Autodesk Fusion 360 part; units mm, degrees
(part 2 of 2)
  line L907 (437.3348, -83.014) -> (451.1912, -83.014)
  line L908 (430.4066, -71.014) -> (437.3348, -83.014)
  line L909 (437.3348, -59.014) -> (430.4066, -71.014)
  line L910 (474.5739, -45.514) -> (460.7175, -45.514)
  line L911 (453.7893, -57.514) -> (460.7175, -69.514)
  line L912 (460.7175, -69.514) -> (474.5739, -69.514)
  line L913 (474.5739, -69.514) -> (481.5021, -57.514)
  line L914 (481.5021, -57.514) -> (474.5739, -45.514)
  line L915 (474.5739, -72.514) -> (460.7175, -72.514)
  line L916 (460.7175, -72.514) -> (453.7893, -84.514)
  line L917 (453.7893, -84.514) -> (460.7175, -96.514)
  line L918 (460.7175, -96.514) -> (474.5739, -96.514)
  line L919 (474.5739, -96.514) -> (481.5021, -84.514)
  line L920 (481.5021, -84.514) -> (474.5739, -72.514)
  line L921 (79.6636, 212.4814) -> (86.5918, 200.4814)
  line L922 (86.5918, 224.4814) -> (79.6636, 212.4814)
  line L923 (100.4482, 224.4814) -> (86.5918, 224.4814)
  line L924 (107.3764, 212.4814) -> (100.4482, 224.4814)
  line L925 (100.4482, 200.4814) -> (107.3764, 212.4814)
  line L926 (109.9745, 210.9814) -> (103.0463, 198.9814)
  line L927 (86.5918, 200.4814) -> (100.4482, 200.4814)
  line L928 (100.4482, 197.4814) -> (86.5918, 197.4814)
  line L929 (107.3764, 185.4814) -> (100.4482, 197.4814)
  line L930 (100.4482, 173.4814) -> (107.3764, 185.4814)
  line L931 (86.5918, 173.4814) -> (100.4482, 173.4814)
  line L932 (79.6636, 185.4814) -> (86.5918, 173.4814)
  line L933 (86.5918, 197.4814) -> (79.6636, 185.4814)
  line L934 (123.8309, 210.9814) -> (109.9745, 210.9814)
  line L935 (103.0463, 198.9814) -> (109.9745, 186.9814)
  line L936 (109.9745, 186.9814) -> (123.8309, 186.9814)
  line L937 (123.8309, 186.9814) -> (130.7591, 198.9814)
  line L938 (130.7591, 198.9814) -> (123.8309, 210.9814)
  line L939 (123.8309, 183.9814) -> (109.9745, 183.9814)
  line L940 (109.9745, 183.9814) -> (103.0463, 171.9814)
  line L941 (103.0463, 171.9814) -> (109.9745, 159.9814)
  line L942 (109.9745, 159.9814) -> (123.8309, 159.9814)
  line L943 (123.8309, 159.9814) -> (130.7591, 171.9814)
  line L944 (130.7591, 171.9814) -> (123.8309, 183.9814)
  line L945 (126.429, 185.4814) -> (133.3572, 173.4814)
  line L946 (133.3572, 197.4814) -> (126.429, 185.4814)
  line L947 (147.2136, 197.4814) -> (133.3572, 197.4814)
  line L948 (154.1418, 185.4814) -> (147.2136, 197.4814)
  line L949 (147.2136, 173.4814) -> (154.1418, 185.4814)
  line L950 (156.7399, 183.9814) -> (149.8117, 171.9814)
  line L951 (133.3572, 173.4814) -> (147.2136, 173.4814)
  line L952 (147.2136, 170.4814) -> (133.3572, 170.4814)
  line L953 (154.1418, 158.4814) -> (147.2136, 170.4814)
  line L954 (147.2136, 146.4814) -> (154.1418, 158.4814)
  line L955 (133.3572, 146.4814) -> (147.2136, 146.4814)
  line L956 (126.429, 158.4814) -> (133.3572, 146.4814)
  line L957 (133.3572, 170.4814) -> (126.429, 158.4814)
  line L958 (170.5963, 183.9814) -> (156.7399, 183.9814)
  line L959 (149.8117, 171.9814) -> (156.7399, 159.9814)
  line L960 (156.7399, 159.9814) -> (170.5963, 159.9814)
  line L961 (170.5963, 159.9814) -> (177.5245, 171.9814)
  line L962 (177.5245, 171.9814) -> (170.5963, 183.9814)
  line L963 (170.5963, 156.9814) -> (156.7399, 156.9814)
  line L964 (156.7399, 156.9814) -> (149.8117, 144.9814)
  line L965 (149.8117, 144.9814) -> (156.7399, 132.9814)
  line L966 (156.7399, 132.9814) -> (170.5963, 132.9814)
  line L967 (170.5963, 132.9814) -> (177.5245, 144.9814)
  line L968 (177.5245, 144.9814) -> (170.5963, 156.9814)
  line L969 (173.1943, 158.4814) -> (180.1225, 146.4814)
  line L970 (180.1225, 170.4814) -> (173.1943, 158.4814)
  line L971 (193.9789, 170.4814) -> (180.1225, 170.4814)
  line L972 (200.9072, 158.4814) -> (193.9789, 170.4814)
  line L973 (193.9789, 146.4814) -> (200.9072, 158.4814)
  line L974 (203.5052, 156.9814) -> (196.577, 144.9814)
  line L975 (180.1225, 146.4814) -> (193.9789, 146.4814)
  line L976 (193.9789, 143.4814) -> (180.1225, 143.4814)
  line L977 (200.9072, 131.4814) -> (193.9789, 143.4814)
  line L978 (193.9789, 119.4814) -> (200.9072, 131.4814)
  line L979 (180.1225, 119.4814) -> (193.9789, 119.4814)
  line L980 (173.1943, 131.4814) -> (180.1225, 119.4814)
  line L981 (180.1225, 143.4814) -> (173.1943, 131.4814)
  line L982 (217.3616, 156.9814) -> (203.5052, 156.9814)
  line L983 (196.577, 144.9814) -> (203.5052, 132.9814)
  line L984 (203.5052, 132.9814) -> (217.3616, 132.9814)
  line L985 (217.3616, 132.9814) -> (224.2898, 144.9814)
  line L986 (224.2898, 144.9814) -> (217.3616, 156.9814)
  line L987 (217.3616, 129.9814) -> (203.5052, 129.9814)
  line L988 (203.5052, 129.9814) -> (196.577, 117.9814)
  line L989 (196.577, 117.9814) -> (203.5052, 105.9814)
  line L990 (203.5052, 105.9814) -> (217.3616, 105.9814)
  line L991 (217.3616, 105.9814) -> (224.2898, 117.9814)
  line L992 (224.2898, 117.9814) -> (217.3616, 129.9814)
  line L993 (219.9597, 131.4814) -> (226.8879, 119.4814)
  line L994 (226.8879, 143.4814) -> (219.9597, 131.4814)
  line L995 (240.7443, 143.4814) -> (226.8879, 143.4814)
  line L996 (247.6725, 131.4814) -> (240.7443, 143.4814)
  line L997 (240.7443, 119.4814) -> (247.6725, 131.4814)
  line L998 (250.2706, 129.9814) -> (243.3424, 117.9814)
  line L999 (226.8879, 119.4814) -> (240.7443, 119.4814)
  line L1000 (240.7443, 116.4814) -> (226.8879, 116.4814)
  line L1001 (247.6725, 104.4814) -> (240.7443, 116.4814)
  line L1002 (240.7443, 92.4814) -> (247.6725, 104.4814)
  line L1003 (226.8879, 92.4814) -> (240.7443, 92.4814)
  line L1004 (219.9597, 104.4814) -> (226.8879, 92.4814)
  line L1005 (226.8879, 116.4814) -> (219.9597, 104.4814)
  line L1006 (264.127, 129.9814) -> (250.2706, 129.9814)
  line L1007 (243.3424, 117.9814) -> (250.2706, 105.9814)
  line L1008 (250.2706, 105.9814) -> (264.127, 105.9814)
  line L1009 (264.127, 105.9814) -> (271.0552, 117.9814)
  line L1010 (271.0552, 117.9814) -> (264.127, 129.9814)
  line L1011 (264.127, 102.9814) -> (250.2706, 102.9814)
  line L1012 (250.2706, 102.9814) -> (243.3424, 90.9814)
  line L1013 (243.3424, 90.9814) -> (250.2706, 78.9814)
  line L1014 (250.2706, 78.9814) -> (264.127, 78.9814)
  line L1015 (264.127, 78.9814) -> (271.0552, 90.9814)
  line L1016 (271.0552, 90.9814) -> (264.127, 102.9814)
  line L1017 (266.7251, 104.4814) -> (273.6533, 92.4814)
  line L1018 (273.6533, 116.4814) -> (266.7251, 104.4814)
  line L1019 (287.5097, 116.4814) -> (273.6533, 116.4814)
  line L1020 (294.4379, 104.4814) -> (287.5097, 116.4814)
  line L1021 (287.5097, 92.4814) -> (294.4379, 104.4814)
  line L1022 (297.036, 102.9814) -> (290.1078, 90.9814)
  line L1023 (273.6533, 92.4814) -> (287.5097, 92.4814)
  line L1024 (287.5097, 89.4814) -> (273.6533, 89.4814)
  line L1025 (294.4379, 77.4814) -> (287.5097, 89.4814)
  line L1026 (287.5097, 65.4814) -> (294.4379, 77.4814)
  line L1027 (273.6533, 65.4814) -> (287.5097, 65.4814)
  line L1028 (266.7251, 77.4814) -> (273.6533, 65.4814)
  line L1029 (273.6533, 89.4814) -> (266.7251, 77.4814)
  line L1030 (310.8924, 102.9814) -> (297.036, 102.9814)
  line L1031 (290.1078, 90.9814) -> (297.036, 78.9814)
  line L1032 (297.036, 78.9814) -> (310.8924, 78.9814)
  line L1033 (310.8924, 78.9814) -> (317.8206, 90.9814)
  line L1034 (317.8206, 90.9814) -> (310.8924, 102.9814)
  line L1035 (310.8924, 75.9814) -> (297.036, 75.9814)
  line L1036 (297.036, 75.9814) -> (290.1078, 63.9814)
  line L1037 (290.1078, 63.9814) -> (297.036, 51.9814)
  line L1038 (297.036, 51.9814) -> (310.8924, 51.9814)
  line L1039 (310.8924, 51.9814) -> (317.8206, 63.9814)
  line L1040 (317.8206, 63.9814) -> (310.8924, 75.9814)
  line L1041 (313.4905, 77.4814) -> (320.4187, 65.4814)
  line L1042 (320.4187, 89.4814) -> (313.4905, 77.4814)
  line L1043 (334.2751, 89.4814) -> (320.4187, 89.4814)
  line L1044 (341.2033, 77.4814) -> (334.2751, 89.4814)
  line L1045 (334.2751, 65.4814) -> (341.2033, 77.4814)
  line L1046 (343.8013, 75.9814) -> (336.8731, 63.9814)
  line L1047 (320.4187, 65.4814) -> (334.2751, 65.4814)
  line L1048 (334.2751, 62.4814) -> (320.4187, 62.4814)
  line L1049 (341.2033, 50.4814) -> (334.2751, 62.4814)
  line L1050 (334.2751, 38.4814) -> (341.2033, 50.4814)
  line L1051 (320.4187, 38.4814) -> (334.2751, 38.4814)
  line L1052 (313.4905, 50.4814) -> (320.4187, 38.4814)
  line L1053 (320.4187, 62.4814) -> (313.4905, 50.4814)
  line L1054 (357.6577, 75.9814) -> (343.8013, 75.9814)
  line L1055 (336.8731, 63.9814) -> (343.8013, 51.9814)
  line L1056 (343.8013, 51.9814) -> (357.6577, 51.9814)
  line L1057 (357.6577, 51.9814) -> (364.586, 63.9814)
  line L1058 (364.586, 63.9814) -> (357.6577, 75.9814)
  line L1059 (357.6577, 48.9814) -> (343.8013, 48.9814)
  line L1060 (343.8013, 48.9814) -> (336.8731, 36.9814)
  line L1061 (336.8731, 36.9814) -> (343.8013, 24.9814)
  line L1062 (343.8013, 24.9814) -> (357.6577, 24.9814)
  line L1063 (357.6577, 24.9814) -> (364.586, 36.9814)
  line L1064 (364.586, 36.9814) -> (357.6577, 48.9814)
  line L1065 (360.2558, 50.4814) -> (367.184, 38.4814)
  line L1066 (367.184, 62.4814) -> (360.2558, 50.4814)
  line L1067 (381.0404, 62.4814) -> (367.184, 62.4814)
  line L1068 (387.9686, 50.4814) -> (381.0404, 62.4814)
  line L1069 (381.0404, 38.4814) -> (387.9686, 50.4814)
  line L1070 (390.5667, 48.9814) -> (383.6385, 36.9814)
  line L1071 (367.184, 38.4814) -> (381.0404, 38.4814)
  line L1072 (381.0404, 35.4814) -> (367.184, 35.4814)
  line L1073 (387.9686, 23.4814) -> (381.0404, 35.4814)
  line L1074 (381.0404, 11.4814) -> (387.9686, 23.4814)
  line L1075 (367.184, 11.4814) -> (381.0404, 11.4814)
  line L1076 (360.2558, 23.4814) -> (367.184, 11.4814)
  line L1077 (367.184, 35.4814) -> (360.2558, 23.4814)
  line L1078 (404.4231, 48.9814) -> (390.5667, 48.9814)
  line L1079 (383.6385, 36.9814) -> (390.5667, 24.9814)
  line L1080 (390.5667, 24.9814) -> (404.4231, 24.9814)
  line L1081 (404.4231, 24.9814) -> (411.3513, 36.9814)
  line L1082 (411.3513, 36.9814) -> (404.4231, 48.9814)
  line L1083 (404.4231, 21.9814) -> (390.5667, 21.9814)
  line L1084 (390.5667, 21.9814) -> (383.6385, 9.9814)
  line L1085 (383.6385, 9.9814) -> (390.5667, -2.0186)
  line L1086 (390.5667, -2.0186) -> (404.4231, -2.0186)
  line L1087 (404.4231, -2.0186) -> (411.3513, 9.9814)
  line L1088 (411.3513, 9.9814) -> (404.4231, 21.9814)
  line L1089 (407.0212, 23.4814) -> (413.9494, 11.4814)
  line L1090 (413.9494, 35.4814) -> (407.0212, 23.4814)
  line L1091 (427.8058, 35.4814) -> (413.9494, 35.4814)
  line L1092 (434.734, 23.4814) -> (427.8058, 35.4814)
  line L1093 (427.8058, 11.4814) -> (434.734, 23.4814)
  line L1094 (437.3321, 21.9814) -> (430.4039, 9.9814)
  line L1095 (413.9494, 11.4814) -> (427.8058, 11.4814)
  line L1096 (427.8058, 8.4814) -> (413.9494, 8.4814)
  line L1097 (434.734, -3.5186) -> (427.8058, 8.4814)
  line L1098 (427.8058, -15.5186) -> (434.734, -3.5186)
  line L1099 (413.9494, -15.5186) -> (427.8058, -15.5186)
  line L1100 (407.0212, -3.5186) -> (413.9494, -15.5186)
  line L1101 (413.9494, 8.4814) -> (407.0212, -3.5186)
  line L1102 (451.1885, 21.9814) -> (437.3321, 21.9814)
  line L1103 (430.4039, 9.9814) -> (437.3321, -2.0186)
  line L1104 (437.3321, -2.0186) -> (451.1885, -2.0186)
  line L1105 (451.1885, -2.0186) -> (458.1167, 9.9814)
  line L1106 (458.1167, 9.9814) -> (451.1885, 21.9814)
  line L1107 (451.1885, -5.0186) -> (437.3321, -5.0186)
  line L1108 (437.3321, -5.0186) -> (430.4039, -17.0186)
  line L1109 (430.4039, -17.0186) -> (437.3321, -29.0186)
  line L1110 (437.3321, -29.0186) -> (451.1885, -29.0186)
  line L1111 (451.1885, -29.0186) -> (458.1167, -17.0186)
  line L1112 (458.1167, -17.0186) -> (451.1885, -5.0186)
  line L1113 (453.7866, -3.5186) -> (460.7148, -15.5186)
  line L1114 (460.7148, 8.4814) -> (453.7866, -3.5186)
  line L1115 (474.5712, 8.4814) -> (460.7148, 8.4814)
  line L1116 (481.4994, -3.5186) -> (474.5712, 8.4814)
  line L1117 (474.5712, -15.5186) -> (481.4994, -3.5186)
  line L1118 (484.0975, -5.0186) -> (477.1693, -17.0186)
  line L1119 (460.7148, -15.5186) -> (474.5712, -15.5186)
  line L1120 (474.5712, -18.5186) -> (460.7148, -18.5186)
  line L1121 (481.4994, -30.5186) -> (474.5712, -18.5186)
  line L1122 (474.5712, -42.5186) -> (481.4994, -30.5186)
  line L1123 (460.7148, -42.5186) -> (474.5712, -42.5186)
  line L1124 (453.7866, -30.5186) -> (460.7148, -42.5186)
  line L1125 (460.7148, -18.5186) -> (453.7866, -30.5186)
  line L1126 (497.9539, -5.0186) -> (484.0975, -5.0186)
  line L1127 (477.1693, -17.0186) -> (484.0975, -29.0186)
  line L1128 (484.0975, -29.0186) -> (497.9539, -29.0186)
  line L1129 (497.9539, -29.0186) -> (504.8821, -17.0186)
  line L1130 (504.8821, -17.0186) -> (497.9539, -5.0186)
  line L1131 (497.9539, -32.0186) -> (484.0975, -32.0186)
  line L1132 (484.0975, -32.0186) -> (477.1693, -44.0186)
  line L1133 (477.1693, -44.0186) -> (484.0975, -56.0186)
  line L1134 (484.0975, -56.0186) -> (497.9539, -56.0186)
  line L1135 (497.9539, -56.0186) -> (504.8821, -44.0186)
  line L1136 (504.8821, -44.0186) -> (497.9539, -32.0186)
  line L1137 (103.0436, 252.9767) -> (109.9718, 240.9767)
  line L1138 (109.9718, 264.9767) -> (103.0436, 252.9767)
  line L1139 (123.8282, 264.9767) -> (109.9718, 264.9767)
  line L1140 (130.7564, 252.9767) -> (123.8282, 264.9767)
  line L1141 (123.8282, 240.9767) -> (130.7564, 252.9767)
  line L1142 (133.3545, 251.4767) -> (126.4263, 239.4767)
  line L1143 (109.9718, 240.9767) -> (123.8282, 240.9767)
  line L1144 (123.8282, 237.9767) -> (109.9718, 237.9767)
  line L1145 (130.7564, 225.9767) -> (123.8282, 237.9767)
  line L1146 (123.8282, 213.9767) -> (130.7564, 225.9767)
  line L1147 (109.9718, 213.9767) -> (123.8282, 213.9767)
  line L1148 (103.0436, 225.9767) -> (109.9718, 213.9767)
  line L1149 (109.9718, 237.9767) -> (103.0436, 225.9767)
  line L1150 (147.2109, 251.4767) -> (133.3545, 251.4767)
  line L1151 (126.4263, 239.4767) -> (133.3545, 227.4767)
  line L1152 (133.3545, 227.4767) -> (147.2109, 227.4767)
  line L1153 (147.2109, 227.4767) -> (154.1391, 239.4767)
  line L1154 (154.1391, 239.4767) -> (147.2109, 251.4767)
  line L1155 (147.2109, 224.4767) -> (133.3545, 224.4767)
  line L1156 (133.3545, 224.4767) -> (126.4263, 212.4767)
  line L1157 (126.4263, 212.4767) -> (133.3545, 200.4767)
  line L1158 (133.3545, 200.4767) -> (147.2109, 200.4767)
  line L1159 (147.2109, 200.4767) -> (154.1391, 212.4767)
  line L1160 (154.1391, 212.4767) -> (147.2109, 224.4767)
  line L1161 (149.809, 225.9767) -> (156.7372, 213.9767)
  line L1162 (156.7372, 237.9767) -> (149.809, 225.9767)
  line L1163 (170.5936, 237.9767) -> (156.7372, 237.9767)
  line L1164 (177.5218, 225.9767) -> (170.5936, 237.9767)
  line L1165 (170.5936, 213.9767) -> (177.5218, 225.9767)
  line L1166 (180.1199, 224.4767) -> (173.1917, 212.4767)
  line L1167 (156.7372, 213.9767) -> (170.5936, 213.9767)
  line L1168 (170.5936, 210.9767) -> (156.7372, 210.9767)
  line L1169 (177.5218, 198.9767) -> (170.5936, 210.9767)
  line L1170 (170.5936, 186.9767) -> (177.5218, 198.9767)
  line L1171 (156.7372, 186.9767) -> (170.5936, 186.9767)
  line L1172 (149.809, 198.9767) -> (156.7372, 186.9767)
  line L1173 (156.7372, 210.9767) -> (149.809, 198.9767)
  line L1174 (193.9763, 224.4767) -> (180.1199, 224.4767)
  line L1175 (173.1917, 212.4767) -> (180.1199, 200.4767)
  line L1176 (180.1199, 200.4767) -> (193.9763, 200.4767)
  line L1177 (193.9763, 200.4767) -> (200.9045, 212.4767)
  line L1178 (200.9045, 212.4767) -> (193.9763, 224.4767)
  line L1179 (193.9763, 197.4767) -> (180.1199, 197.4767)
  line L1180 (180.1199, 197.4767) -> (173.1917, 185.4767)
  line L1181 (173.1917, 185.4767) -> (180.1199, 173.4767)
  line L1182 (180.1199, 173.4767) -> (193.9763, 173.4767)
  line L1183 (193.9763, 173.4767) -> (200.9045, 185.4767)
  line L1184 (200.9045, 185.4767) -> (193.9763, 197.4767)
  line L1185 (196.5743, 198.9767) -> (203.5025, 186.9767)
  line L1186 (203.5025, 210.9767) -> (196.5743, 198.9767)
  line L1187 (217.3589, 210.9767) -> (203.5025, 210.9767)
  line L1188 (224.2872, 198.9767) -> (217.3589, 210.9767)
  line L1189 (217.3589, 186.9767) -> (224.2872, 198.9767)
  line L1190 (226.8852, 197.4767) -> (219.957, 185.4767)
  line L1191 (203.5025, 186.9767) -> (217.3589, 186.9767)
  line L1192 (217.3589, 183.9767) -> (203.5025, 183.9767)
  line L1193 (224.2872, 171.9767) -> (217.3589, 183.9767)
  line L1194 (217.3589, 159.9767) -> (224.2872, 171.9767)
  line L1195 (203.5025, 159.9767) -> (217.3589, 159.9767)
  line L1196 (196.5743, 171.9767) -> (203.5025, 159.9767)
  line L1197 (203.5025, 183.9767) -> (196.5743, 171.9767)
  line L1198 (240.7416, 197.4767) -> (226.8852, 197.4767)
  line L1199 (219.957, 185.4767) -> (226.8852, 173.4767)
  line L1200 (226.8852, 173.4767) -> (240.7416, 173.4767)
  line L1201 (240.7416, 173.4767) -> (247.6698, 185.4767)
  line L1202 (247.6698, 185.4767) -> (240.7416, 197.4767)
  line L1203 (240.7416, 170.4767) -> (226.8852, 170.4767)
  line L1204 (226.8852, 170.4767) -> (219.957, 158.4767)
  line L1205 (219.957, 158.4767) -> (226.8852, 146.4767)
  line L1206 (226.8852, 146.4767) -> (240.7416, 146.4767)
  line L1207 (240.7416, 146.4767) -> (247.6698, 158.4767)
  line L1208 (247.6698, 158.4767) -> (240.7416, 170.4767)
  line L1209 (243.3397, 171.9767) -> (250.2679, 159.9767)
  line L1210 (250.2679, 183.9767) -> (243.3397, 171.9767)
  line L1211 (264.1243, 183.9767) -> (250.2679, 183.9767)
  line L1212 (271.0525, 171.9767) -> (264.1243, 183.9767)
  line L1213 (264.1243, 159.9767) -> (271.0525, 171.9767)
  line L1214 (273.6506, 170.4767) -> (266.7224, 158.4767)
  line L1215 (250.2679, 159.9767) -> (264.1243, 159.9767)
  line L1216 (264.1243, 156.9767) -> (250.2679, 156.9767)
  line L1217 (271.0525, 144.9767) -> (264.1243, 156.9767)
  line L1218 (264.1243, 132.9767) -> (271.0525, 144.9767)
  line L1219 (250.2679, 132.9767) -> (264.1243, 132.9767)
  line L1220 (243.3397, 144.9767) -> (250.2679, 132.9767)
  line L1221 (250.2679, 156.9767) -> (243.3397, 144.9767)
  line L1222 (287.507, 170.4767) -> (273.6506, 170.4767)
  line L1223 (266.7224, 158.4767) -> (273.6506, 146.4767)
  line L1224 (273.6506, 146.4767) -> (287.507, 146.4767)
  line L1225 (287.507, 146.4767) -> (294.4352, 158.4767)
  line L1226 (294.4352, 158.4767) -> (287.507, 170.4767)
  line L1227 (287.507, 143.4767) -> (273.6506, 143.4767)
  line L1228 (273.6506, 143.4767) -> (266.7224, 131.4767)
  line L1229 (266.7224, 131.4767) -> (273.6506, 119.4767)
  line L1230 (273.6506, 119.4767) -> (287.507, 119.4767)
  line L1231 (287.507, 119.4767) -> (294.4352, 131.4767)
  line L1232 (294.4352, 131.4767) -> (287.507, 143.4767)
  line L1233 (290.1051, 144.9767) -> (297.0333, 132.9767)
  line L1234 (297.0333, 156.9767) -> (290.1051, 144.9767)
  line L1235 (310.8897, 156.9767) -> (297.0333, 156.9767)
  line L1236 (317.8179, 144.9767) -> (310.8897, 156.9767)
  line L1237 (310.8897, 132.9767) -> (317.8179, 144.9767)
  line L1238 (320.416, 143.4767) -> (313.4878, 131.4767)
  line L1239 (297.0333, 132.9767) -> (310.8897, 132.9767)
  line L1240 (310.8897, 129.9767) -> (297.0333, 129.9767)
  line L1241 (317.8179, 117.9767) -> (310.8897, 129.9767)
  line L1242 (310.8897, 105.9767) -> (317.8179, 117.9767)
  line L1243 (297.0333, 105.9767) -> (310.8897, 105.9767)
  line L1244 (290.1051, 117.9767) -> (297.0333, 105.9767)
  line L1245 (297.0333, 129.9767) -> (290.1051, 117.9767)
  line L1246 (334.2724, 143.4767) -> (320.416, 143.4767)
  line L1247 (313.4878, 131.4767) -> (320.416, 119.4767)
  line L1248 (320.416, 119.4767) -> (334.2724, 119.4767)
  line L1249 (334.2724, 119.4767) -> (341.2006, 131.4767)
  line L1250 (341.2006, 131.4767) -> (334.2724, 143.4767)
  line L1251 (334.2724, 116.4767) -> (320.416, 116.4767)
  line L1252 (320.416, 116.4767) -> (313.4878, 104.4767)
  line L1253 (313.4878, 104.4767) -> (320.416, 92.4767)
  line L1254 (320.416, 92.4767) -> (334.2724, 92.4767)
  line L1255 (334.2724, 92.4767) -> (341.2006, 104.4767)
  line L1256 (341.2006, 104.4767) -> (334.2724, 116.4767)
  line L1257 (336.8705, 117.9767) -> (343.7987, 105.9767)
  line L1258 (343.7987, 129.9767) -> (336.8705, 117.9767)
  line L1259 (357.6551, 129.9767) -> (343.7987, 129.9767)
  line L1260 (364.5833, 117.9767) -> (357.6551, 129.9767)
  line L1261 (357.6551, 105.9767) -> (364.5833, 117.9767)
  line L1262 (367.1813, 116.4767) -> (360.2531, 104.4767)
  line L1263 (343.7987, 105.9767) -> (357.6551, 105.9767)
  line L1264 (357.6551, 102.9767) -> (343.7987, 102.9767)
  line L1265 (364.5833, 90.9767) -> (357.6551, 102.9767)
  line L1266 (357.6551, 78.9767) -> (364.5833, 90.9767)
  line L1267 (343.7987, 78.9767) -> (357.6551, 78.9767)
  line L1268 (336.8705, 90.9767) -> (343.7987, 78.9767)
  line L1269 (343.7987, 102.9767) -> (336.8705, 90.9767)
  line L1270 (381.0377, 116.4767) -> (367.1813, 116.4767)
  line L1271 (360.2531, 104.4767) -> (367.1813, 92.4767)
  line L1272 (367.1813, 92.4767) -> (381.0377, 92.4767)
  line L1273 (381.0377, 92.4767) -> (387.966, 104.4767)
  line L1274 (387.966, 104.4767) -> (381.0377, 116.4767)
  line L1275 (381.0377, 89.4767) -> (367.1813, 89.4767)
  line L1276 (367.1813, 89.4767) -> (360.2531, 77.4767)
  line L1277 (360.2531, 77.4767) -> (367.1813, 65.4767)
  line L1278 (367.1813, 65.4767) -> (381.0377, 65.4767)
  line L1279 (381.0377, 65.4767) -> (387.966, 77.4767)
  line L1280 (387.966, 77.4767) -> (381.0377, 89.4767)
  line L1281 (383.6358, 90.9767) -> (390.564, 78.9767)
  line L1282 (390.564, 102.9767) -> (383.6358, 90.9767)
  line L1283 (404.4204, 102.9767) -> (390.564, 102.9767)
  line L1284 (411.3486, 90.9767) -> (404.4204, 102.9767)
  line L1285 (404.4204, 78.9767) -> (411.3486, 90.9767)
  line L1286 (413.9467, 89.4767) -> (407.0185, 77.4767)
  line L1287 (390.564, 78.9767) -> (404.4204, 78.9767)
  line L1288 (404.4204, 75.9767) -> (390.564, 75.9767)
  line L1289 (411.3486, 63.9767) -> (404.4204, 75.9767)
  line L1290 (404.4204, 51.9767) -> (411.3486, 63.9767)
  line L1291 (390.564, 51.9767) -> (404.4204, 51.9767)
  line L1292 (383.6358, 63.9767) -> (390.564, 51.9767)
  line L1293 (390.564, 75.9767) -> (383.6358, 63.9767)
  line L1294 (427.8031, 89.4767) -> (413.9467, 89.4767)
  line L1295 (407.0185, 77.4767) -> (413.9467, 65.4767)
  line L1296 (413.9467, 65.4767) -> (427.8031, 65.4767)
  line L1297 (427.8031, 65.4767) -> (434.7313, 77.4767)
  line L1298 (434.7313, 77.4767) -> (427.8031, 89.4767)
  line L1299 (427.8031, 62.4767) -> (413.9467, 62.4767)
  line L1300 (413.9467, 62.4767) -> (407.0185, 50.4767)
  line L1301 (407.0185, 50.4767) -> (413.9467, 38.4767)
  line L1302 (413.9467, 38.4767) -> (427.8031, 38.4767)
  line L1303 (427.8031, 38.4767) -> (434.7313, 50.4767)
  line L1304 (434.7313, 50.4767) -> (427.8031, 62.4767)
  line L1305 (430.4012, 63.9767) -> (437.3294, 51.9767)
  line L1306 (437.3294, 75.9767) -> (430.4012, 63.9767)
  line L1307 (451.1858, 75.9767) -> (437.3294, 75.9767)
  line L1308 (458.114, 63.9767) -> (451.1858, 75.9767)
  line L1309 (451.1858, 51.9767) -> (458.114, 63.9767)
  line L1310 (460.7121, 62.4767) -> (453.7839, 50.4767)
  line L1311 (437.3294, 51.9767) -> (451.1858, 51.9767)
  line L1312 (451.1858, 48.9767) -> (437.3294, 48.9767)
  line L1313 (458.114, 36.9767) -> (451.1858, 48.9767)
  line L1314 (451.1858, 24.9767) -> (458.114, 36.9767)
  line L1315 (437.3294, 24.9767) -> (451.1858, 24.9767)
  line L1316 (430.4012, 36.9767) -> (437.3294, 24.9767)
  line L1317 (437.3294, 48.9767) -> (430.4012, 36.9767)
  line L1318 (474.5685, 62.4767) -> (460.7121, 62.4767)
  line L1319 (453.7839, 50.4767) -> (460.7121, 38.4767)
  line L1320 (460.7121, 38.4767) -> (474.5685, 38.4767)
  line L1321 (474.5685, 38.4767) -> (481.4967, 50.4767)
  line L1322 (481.4967, 50.4767) -> (474.5685, 62.4767)
  line L1323 (474.5685, 35.4767) -> (460.7121, 35.4767)
  line L1324 (460.7121, 35.4767) -> (453.7839, 23.4767)
  line L1325 (453.7839, 23.4767) -> (460.7121, 11.4767)
  line L1326 (460.7121, 11.4767) -> (474.5685, 11.4767)
  line L1327 (474.5685, 11.4767) -> (481.4967, 23.4767)
  line L1328 (481.4967, 23.4767) -> (474.5685, 35.4767)
  line L1329 (477.1666, 36.9767) -> (484.0948, 24.9767)
  line L1330 (484.0948, 48.9767) -> (477.1666, 36.9767)
  line L1331 (497.9512, 48.9767) -> (484.0948, 48.9767)
  line L1332 (504.8794, 36.9767) -> (497.9512, 48.9767)
  line L1333 (497.9512, 24.9767) -> (504.8794, 36.9767)
  line L1334 (507.4775, 35.4767) -> (500.5493, 23.4767)
  line L1335 (484.0948, 24.9767) -> (497.9512, 24.9767)
  line L1336 (497.9512, 21.9767) -> (484.0948, 21.9767)
  line L1337 (504.8794, 9.9767) -> (497.9512, 21.9767)
  line L1338 (497.9512, -2.0233) -> (504.8794, 9.9767)
  line L1339 (484.0948, -2.0233) -> (497.9512, -2.0233)
  line L1340 (477.1666, 9.9767) -> (484.0948, -2.0233)
  line L1341 (484.0948, 21.9767) -> (477.1666, 9.9767)
  line L1342 (521.3339, 35.4767) -> (507.4775, 35.4767)
  line L1343 (500.5493, 23.4767) -> (507.4775, 11.4767)
  line L1344 (507.4775, 11.4767) -> (521.3339, 11.4767)
  line L1345 (521.3339, 11.4767) -> (528.2621, 23.4767)
  line L1346 (528.2621, 23.4767) -> (521.3339, 35.4767)
  line L1347 (521.3339, 8.4767) -> (507.4775, 8.4767)
  line L1348 (507.4775, 8.4767) -> (500.5493, -3.5233)
  line L1349 (500.5493, -3.5233) -> (507.4775, -15.5233)
  line L1350 (507.4775, -15.5233) -> (521.3339, -15.5233)
  line L1351 (521.3339, -15.5233) -> (528.2621, -3.5233)
  line L1352 (528.2621, -3.5233) -> (521.3339, 8.4767)
  line L1353 (126.4236, 293.4721) -> (133.3518, 281.4721)
  line L1354 (133.3518, 305.4721) -> (126.4236, 293.4721)
  line L1355 (147.2082, 305.4721) -> (133.3518, 305.4721)
  line L1356 (154.1364, 293.4721) -> (147.2082, 305.4721)
  line L1357 (147.2082, 281.4721) -> (154.1364, 293.4721)
  line L1358 (156.7345, 291.9721) -> (149.8063, 279.9721)
  line L1359 (133.3518, 281.4721) -> (147.2082, 281.4721)
  line L1360 (147.2082, 278.4721) -> (133.3518, 278.4721)
  line L1361 (154.1364, 266.4721) -> (147.2082, 278.4721)
  line L1362 (147.2082, 254.4721) -> (154.1364, 266.4721)
  line L1363 (133.3518, 254.4721) -> (147.2082, 254.4721)
  line L1364 (126.4236, 266.4721) -> (133.3518, 254.4721)
  line L1365 (133.3518, 278.4721) -> (126.4236, 266.4721)
  line L1366 (170.5909, 291.9721) -> (156.7345, 291.9721)
  line L1367 (149.8063, 279.9721) -> (156.7345, 267.9721)
  line L1368 (156.7345, 267.9721) -> (170.5909, 267.9721)
  line L1369 (170.5909, 267.9721) -> (177.5191, 279.9721)
  line L1370 (177.5191, 279.9721) -> (170.5909, 291.9721)
  line L1371 (170.5909, 264.9721) -> (156.7345, 264.9721)
  line L1372 (156.7345, 264.9721) -> (149.8063, 252.9721)
  line L1373 (149.8063, 252.9721) -> (156.7345, 240.9721)
  line L1374 (156.7345, 240.9721) -> (170.5909, 240.9721)
  line L1375 (170.5909, 240.9721) -> (177.5191, 252.9721)
  line L1376 (177.5191, 252.9721) -> (170.5909, 264.9721)
  line L1377 (173.189, 266.4721) -> (180.1172, 254.4721)
  line L1378 (180.1172, 278.4721) -> (173.189, 266.4721)
  line L1379 (193.9736, 278.4721) -> (180.1172, 278.4721)
  line L1380 (200.9018, 266.4721) -> (193.9736, 278.4721)
  line L1381 (193.9736, 254.4721) -> (200.9018, 266.4721)
  line L1382 (203.4999, 264.9721) -> (196.5717, 252.9721)
  line L1383 (180.1172, 254.4721) -> (193.9736, 254.4721)
  line L1384 (193.9736, 251.4721) -> (180.1172, 251.4721)
  line L1385 (200.9018, 239.4721) -> (193.9736, 251.4721)
  line L1386 (193.9736, 227.4721) -> (200.9018, 239.4721)
  line L1387 (180.1172, 227.4721) -> (193.9736, 227.4721)
  line L1388 (173.189, 239.4721) -> (180.1172, 227.4721)
  line L1389 (180.1172, 251.4721) -> (173.189, 239.4721)
  line L1390 (217.3563, 264.9721) -> (203.4999, 264.9721)
  line L1391 (196.5717, 252.9721) -> (203.4999, 240.9721)
  line L1392 (203.4999, 240.9721) -> (217.3563, 240.9721)
  line L1393 (217.3563, 240.9721) -> (224.2845, 252.9721)
  line L1394 (224.2845, 252.9721) -> (217.3563, 264.9721)
  line L1395 (217.3563, 237.9721) -> (203.4999, 237.9721)
  line L1396 (203.4999, 237.9721) -> (196.5717, 225.9721)
  line L1397 (196.5717, 225.9721) -> (203.4999, 213.9721)
  line L1398 (203.4999, 213.9721) -> (217.3563, 213.9721)
  line L1399 (217.3563, 213.9721) -> (224.2845, 225.9721)
  line L1400 (224.2845, 225.9721) -> (217.3563, 237.9721)
  line L1401 (219.9543, 239.4721) -> (226.8825, 227.4721)
  line L1402 (226.8825, 251.4721) -> (219.9543, 239.4721)
  line L1403 (240.7389, 251.4721) -> (226.8825, 251.4721)
  line L1404 (247.6672, 239.4721) -> (240.7389, 251.4721)
  line L1405 (240.7389, 227.4721) -> (247.6672, 239.4721)
  line L1406 (250.2652, 237.9721) -> (243.337, 225.9721)
  line L1407 (226.8825, 227.4721) -> (240.7389, 227.4721)
  line L1408 (240.7389, 224.4721) -> (226.8825, 224.4721)
  line L1409 (247.6672, 212.4721) -> (240.7389, 224.4721)
  line L1410 (240.7389, 200.4721) -> (247.6672, 212.4721)
  line L1411 (226.8825, 200.4721) -> (240.7389, 200.4721)
  line L1412 (219.9543, 212.4721) -> (226.8825, 200.4721)
  line L1413 (226.8825, 224.4721) -> (219.9543, 212.4721)
  line L1414 (264.1216, 237.9721) -> (250.2652, 237.9721)
  line L1415 (243.337, 225.9721) -> (250.2652, 213.9721)
  line L1416 (250.2652, 213.9721) -> (264.1216, 213.9721)
  line L1417 (264.1216, 213.9721) -> (271.0498, 225.9721)
  line L1418 (271.0498, 225.9721) -> (264.1216, 237.9721)
  line L1419 (264.1216, 210.9721) -> (250.2652, 210.9721)
  line L1420 (250.2652, 210.9721) -> (243.337, 198.9721)
  line L1421 (243.337, 198.9721) -> (250.2652, 186.9721)
  line L1422 (250.2652, 186.9721) -> (264.1216, 186.9721)
  line L1423 (264.1216, 186.9721) -> (271.0498, 198.9721)
  line L1424 (271.0498, 198.9721) -> (264.1216, 210.9721)
  line L1425 (266.7197, 212.4721) -> (273.6479, 200.4721)
  line L1426 (273.6479, 224.4721) -> (266.7197, 212.4721)
  line L1427 (287.5043, 224.4721) -> (273.6479, 224.4721)
  line L1428 (294.4325, 212.4721) -> (287.5043, 224.4721)
  line L1429 (287.5043, 200.4721) -> (294.4325, 212.4721)
  line L1430 (297.0306, 210.9721) -> (290.1024, 198.9721)
  line L1431 (273.6479, 200.4721) -> (287.5043, 200.4721)
  line L1432 (287.5043, 197.4721) -> (273.6479, 197.4721)
  line L1433 (294.4325, 185.4721) -> (287.5043, 197.4721)
  line L1434 (287.5043, 173.4721) -> (294.4325, 185.4721)
  line L1435 (273.6479, 173.4721) -> (287.5043, 173.4721)
  line L1436 (266.7197, 185.4721) -> (273.6479, 173.4721)
  line L1437 (273.6479, 197.4721) -> (266.7197, 185.4721)
  line L1438 (310.887, 210.9721) -> (297.0306, 210.9721)
  line L1439 (290.1024, 198.9721) -> (297.0306, 186.9721)
  line L1440 (297.0306, 186.9721) -> (310.887, 186.9721)
  line L1441 (310.887, 186.9721) -> (317.8152, 198.9721)
  line L1442 (317.8152, 198.9721) -> (310.887, 210.9721)
  line L1443 (310.887, 183.9721) -> (297.0306, 183.9721)
  line L1444 (297.0306, 183.9721) -> (290.1024, 171.9721)
  line L1445 (290.1024, 171.9721) -> (297.0306, 159.9721)
  line L1446 (297.0306, 159.9721) -> (310.887, 159.9721)
  line L1447 (310.887, 159.9721) -> (317.8152, 171.9721)
  line L1448 (317.8152, 171.9721) -> (310.887, 183.9721)
  line L1449 (313.4851, 185.4721) -> (320.4133, 173.4721)
  line L1450 (320.4133, 197.4721) -> (313.4851, 185.4721)
  line L1451 (334.2697, 197.4721) -> (320.4133, 197.4721)
  line L1452 (341.1979, 185.4721) -> (334.2697, 197.4721)
  line L1453 (334.2697, 173.4721) -> (341.1979, 185.4721)
  line L1454 (343.796, 183.9721) -> (336.8678, 171.9721)
  line L1455 (320.4133, 173.4721) -> (334.2697, 173.4721)
  line L1456 (334.2697, 170.4721) -> (320.4133, 170.4721)
  line L1457 (341.1979, 158.4721) -> (334.2697, 170.4721)
  line L1458 (334.2697, 146.4721) -> (341.1979, 158.4721)
  line L1459 (320.4133, 146.4721) -> (334.2697, 146.4721)
  line L1460 (313.4851, 158.4721) -> (320.4133, 146.4721)
  line L1461 (320.4133, 170.4721) -> (313.4851, 158.4721)
  line L1462 (357.6524, 183.9721) -> (343.796, 183.9721)
  line L1463 (336.8678, 171.9721) -> (343.796, 159.9721)
  line L1464 (343.796, 159.9721) -> (357.6524, 159.9721)
  line L1465 (357.6524, 159.9721) -> (364.5806, 171.9721)
  line L1466 (364.5806, 171.9721) -> (357.6524, 183.9721)
  line L1467 (357.6524, 156.9721) -> (343.796, 156.9721)
  line L1468 (343.796, 156.9721) -> (336.8678, 144.9721)
  line L1469 (336.8678, 144.9721) -> (343.796, 132.9721)
  line L1470 (343.796, 132.9721) -> (357.6524, 132.9721)
  line L1471 (357.6524, 132.9721) -> (364.5806, 144.9721)
  line L1472 (364.5806, 144.9721) -> (357.6524, 156.9721)
  line L1473 (360.2505, 158.4721) -> (367.1787, 146.4721)
  line L1474 (367.1787, 170.4721) -> (360.2505, 158.4721)
  line L1475 (381.0351, 170.4721) -> (367.1787, 170.4721)
  line L1476 (387.9633, 158.4721) -> (381.0351, 170.4721)
  line L1477 (381.0351, 146.4721) -> (387.9633, 158.4721)
  line L1478 (390.5613, 156.9721) -> (383.6331, 144.9721)
  line L1479 (367.1787, 146.4721) -> (381.0351, 146.4721)
  line L1480 (381.0351, 143.4721) -> (367.1787, 143.4721)
  line L1481 (387.9633, 131.4721) -> (381.0351, 143.4721)
  line L1482 (381.0351, 119.4721) -> (387.9633, 131.4721)
  line L1483 (367.1787, 119.4721) -> (381.0351, 119.4721)
  line L1484 (360.2505, 131.4721) -> (367.1787, 119.4721)
  line L1485 (367.1787, 143.4721) -> (360.2505, 131.4721)
  line L1486 (404.4177, 156.9721) -> (390.5613, 156.9721)
  line L1487 (383.6331, 144.9721) -> (390.5613, 132.9721)
  line L1488 (390.5613, 132.9721) -> (404.4177, 132.9721)
  line L1489 (404.4177, 132.9721) -> (411.346, 144.9721)
  line L1490 (411.346, 144.9721) -> (404.4177, 156.9721)
  line L1491 (404.4177, 129.9721) -> (390.5613, 129.9721)
  line L1492 (390.5613, 129.9721) -> (383.6331, 117.9721)
  line L1493 (383.6331, 117.9721) -> (390.5613, 105.9721)
  line L1494 (390.5613, 105.9721) -> (404.4177, 105.9721)
  line L1495 (404.4177, 105.9721) -> (411.346, 117.9721)
  line L1496 (411.346, 117.9721) -> (404.4177, 129.9721)
  line L1497 (407.0158, 131.4721) -> (413.944, 119.4721)
  line L1498 (413.944, 143.4721) -> (407.0158, 131.4721)
  line L1499 (427.8004, 143.4721) -> (413.944, 143.4721)
  line L1500 (434.7286, 131.4721) -> (427.8004, 143.4721)
  line L1501 (427.8004, 119.4721) -> (434.7286, 131.4721)
  line L1502 (437.3267, 129.9721) -> (430.3985, 117.9721)
  line L1503 (413.944, 119.4721) -> (427.8004, 119.4721)
  line L1504 (427.8004, 116.4721) -> (413.944, 116.4721)
  line L1505 (434.7286, 104.4721) -> (427.8004, 116.4721)
  line L1506 (427.8004, 92.4721) -> (434.7286, 104.4721)
  line L1507 (413.944, 92.4721) -> (427.8004, 92.4721)
  line L1508 (407.0158, 104.4721) -> (413.944, 92.4721)
  line L1509 (413.944, 116.4721) -> (407.0158, 104.4721)
  line L1510 (451.1831, 129.9721) -> (437.3267, 129.9721)
  line L1511 (430.3985, 117.9721) -> (437.3267, 105.9721)
  line L1512 (437.3267, 105.9721) -> (451.1831, 105.9721)
  line L1513 (451.1831, 105.9721) -> (458.1113, 117.9721)
  line L1514 (458.1113, 117.9721) -> (451.1831, 129.9721)
  line L1515 (451.1831, 102.9721) -> (437.3267, 102.9721)
  line L1516 (437.3267, 102.9721) -> (430.3985, 90.9721)
  line L1517 (430.3985, 90.9721) -> (437.3267, 78.9721)
  line L1518 (437.3267, 78.9721) -> (451.1831, 78.9721)
  line L1519 (451.1831, 78.9721) -> (458.1113, 90.9721)
  line L1520 (458.1113, 90.9721) -> (451.1831, 102.9721)
  line L1521 (453.7812, 104.4721) -> (460.7094, 92.4721)
  line L1522 (460.7094, 116.4721) -> (453.7812, 104.4721)
  line L1523 (474.5658, 116.4721) -> (460.7094, 116.4721)
  line L1524 (481.494, 104.4721) -> (474.5658, 116.4721)
  line L1525 (474.5658, 92.4721) -> (481.494, 104.4721)
  line L1526 (484.0921, 102.9721) -> (477.1639, 90.9721)
  line L1527 (460.7094, 92.4721) -> (474.5658, 92.4721)
  line L1528 (474.5658, 89.4721) -> (460.7094, 89.4721)
  line L1529 (481.494, 77.4721) -> (474.5658, 89.4721)
  line L1530 (474.5658, 65.4721) -> (481.494, 77.4721)
  line L1531 (460.7094, 65.4721) -> (474.5658, 65.4721)
  line L1532 (453.7812, 77.4721) -> (460.7094, 65.4721)
  line L1533 (460.7094, 89.4721) -> (453.7812, 77.4721)
  line L1534 (497.9485, 102.9721) -> (484.0921, 102.9721)
  line L1535 (477.1639, 90.9721) -> (484.0921, 78.9721)
  line L1536 (484.0921, 78.9721) -> (497.9485, 78.9721)
  line L1537 (497.9485, 78.9721) -> (504.8767, 90.9721)
  line L1538 (504.8767, 90.9721) -> (497.9485, 102.9721)
  line L1539 (497.9485, 75.9721) -> (484.0921, 75.9721)
  line L1540 (484.0921, 75.9721) -> (477.1639, 63.9721)
  line L1541 (477.1639, 63.9721) -> (484.0921, 51.9721)
  line L1542 (484.0921, 51.9721) -> (497.9485, 51.9721)
  line L1543 (497.9485, 51.9721) -> (504.8767, 63.9721)
  line L1544 (504.8767, 63.9721) -> (497.9485, 75.9721)
  line L1545 (500.5466, 77.4721) -> (507.4748, 65.4721)
  line L1546 (507.4748, 89.4721) -> (500.5466, 77.4721)
  line L1547 (521.3312, 89.4721) -> (507.4748, 89.4721)
  line L1548 (528.2594, 77.4721) -> (521.3312, 89.4721)
  line L1549 (521.3312, 65.4721) -> (528.2594, 77.4721)
  line L1550 (530.8575, 75.9721) -> (523.9293, 63.9721)
  line L1551 (507.4748, 65.4721) -> (521.3312, 65.4721)
  line L1552 (521.3312, 62.4721) -> (507.4748, 62.4721)
  line L1553 (528.2594, 50.4721) -> (521.3312, 62.4721)
  line L1554 (521.3312, 38.4721) -> (528.2594, 50.4721)
  line L1555 (507.4748, 38.4721) -> (521.3312, 38.4721)
  line L1556 (500.5466, 50.4721) -> (507.4748, 38.4721)
  line L1557 (507.4748, 62.4721) -> (500.5466, 50.4721)
  line L1558 (544.7139, 75.9721) -> (530.8575, 75.9721)
  line L1559 (523.9293, 63.9721) -> (530.8575, 51.9721)
  line L1560 (530.8575, 51.9721) -> (544.7139, 51.9721)
  line L1561 (544.7139, 51.9721) -> (551.6421, 63.9721)
  line L1562 (551.6421, 63.9721) -> (544.7139, 75.9721)
  line L1563 (544.7139, 48.9721) -> (530.8575, 48.9721)
  line L1564 (530.8575, 48.9721) -> (523.9293, 36.9721)
  line L1565 (523.9293, 36.9721) -> (530.8575, 24.9721)
  line L1566 (530.8575, 24.9721) -> (544.7139, 24.9721)
  line L1567 (544.7139, 24.9721) -> (551.6421, 36.9721)
  line L1568 (551.6421, 36.9721) -> (544.7139, 48.9721)
  point P0 (340, 0)
  point P1 (150, 99.7133)
  point P2 (0, 50.5)
  point P3 (23.3827, 37)
  point P4 (0, 23.5)
  point P5 (23.3827, 10)
  point P6 (23.3827, 37)
  point P7 (0, 50.5)
  point P8 (23.3827, 37)
  point P9 (0, 23.5)
  point P10 (23.3827, 10)
  point P11 (0, 77.5)
  point P12 (137.5, 146)
  dimension "d1" = 490
  dimension "d10" = 20
  dimension "d11" = 20
  dimension "d12" = 20
  dimension "d13" = 20
  dimension "d16" = 4.35
  dimension "d17" = 6
  dimension "d18" = 6
  dimension "d23" = 40
  dimension "d24" = -101
  dimension "d26" = 30
  dimension "d28" = 27
  dimension "d29" = 150
  dimension "d31" = 30
  dimension "d32" = 27
  dimension "d34" = 27
  dimension "d43" = 6
  dimension "d44" = 6
  dimension "d45" = 6
  dimension "d46" = 6
  dimension "d48" = 10
  dimension "d49" = 10
  dimension "d50" = 10
  dimension "d51" = 10
  dimension "d65" = 5
  dimension "d66" = 2.5
  dimension "d67" = 2.5
  dimension "d68" = -2.5
  dimension "d69" = 2.5
  dimension "d70" = 2.5
  dimension "d71" = 2.5
  dimension "d72" = 2.5
  dimension "d78" = 23.3827
  dimension "d79" = 12
  dimension "d80" = 12
  dimension "d81" = 12
  dimension "d82" = 12
  dimension "d85" = 54
  dimension "d86" = 46.76
  dimension "d87" = 12
  dimension "d88" = 27
  dimension "d89" = 3
  dimension "d90" = -3
  dimension "d91" = 15
  dimension "d92" = 30
  dimension "d93" = 40
  dimension "d94" = 30
  dimension "d95" = 5
  dimension "d96" = 240
  dimension "d97" = 245
  dimension "d98" = 30
  dimension "d99" = 10
  dimension "d100" = 30
  constraint horizontal L0
  constraint vertical L1
  constraint horizontal L2
  constraint vertical L3
  constraint coincident L0.start L3.end
  constraint coincident L2.end L3.start
  constraint coincident L1.end L2.start
  constraint coincident L0.end L1.start
  constraint coincident L0 P0
  constraint midpoint L3 P7
  constraint midpoint L1 L4.end
  constraint coincident A0 L15.start
  constraint coincident A2 L16.end
  constraint parallel L2 L15
  constraint coincident A3 L17.start
  constraint coincident A1 L18.end
  constraint parallel L0 L17
  constraint concentric A4 A5
  constraint tangent A5 L15
  constraint coincident P7 P2
  constraint horizontal L6
  constraint coincident P8 P6
  constraint horizontal L8
  constraint coincident L3 P9
  constraint coincident P9 P4
  constraint horizontal L10
  constraint coincident P10 P5
  constraint perpendicular L14 L17
  constraint concentric A1 A6
  constraint concentric A0 A7
  constraint concentric A3 A8
  constraint concentric A2 A9
  constraint collinear L15 L16
  constraint collinear L17 L18
  constraint tangent L13 A10
  constraint tangent L20 A10
  constraint tangent L11 A11
  constraint tangent L19 A11
  constraint tangent L19 A12
  constraint tangent L14 A12
  constraint tangent L20 A13
  constraint tangent L12 A13
  constraint tangent L13 A16
  constraint coincident L13.start A16
  constraint coincident L15.end A16
  constraint vertical L12
  constraint tangent L12 A30
  constraint coincident L12.start A30
  constraint coincident L18.start A30
  constraint vertical L11
  constraint coincident L11.start A18
  constraint coincident L16.start A18
  constraint horizontal L19
  constraint horizontal L20
  constraint vertical L13
  constraint coincident L14.end A32
  constraint tangent L14 A32
  constraint horizontal L36
  constraint horizontal L48
  constraint horizontal L39
  constraint horizontal L54
  constraint coincident L3 P11
  constraint horizontal L60
  constraint coincident A7 L61.start
  constraint coincident L2 L61.start
  constraint coincident A6 L61.end
  constraint coincident L0 L61.end
  constraint coincident A9 L62.start
  constraint coincident L2 L62.start
  constraint coincident A8 L62.end
  constraint coincident L0 L62.end
  constraint coincident L17.end A32
  constraint coincident A4.centre A5.centre
  constraint perpendicular L27 L65
  constraint horizontal L66
  constraint perpendicular L66 L67
  constraint parallel L66 L68
  constraint parallel L67 L69
  constraint coincident L70 P12
  constraint coincident L71 P12
  constraint coincident P12 L65.end
  constraint horizontal L72
  constraint vertical L73
  constraint horizontal L74
  constraint vertical L75
  constraint horizontal L76
  constraint vertical L77
  constraint horizontal L78
  constraint vertical L79
  constraint midpoint L76 L80.start
  constraint midpoint L78 L80.end
  constraint collinear L75 L79
  constraint coincident L2 A4.centre
  constraint tangent L11 A18
  constraint collinear L66 L74
  constraint tangent L18 A30
  measures "d1" distance of L0.start L0.end
  measures "d10" diameter of A0
  measures "d11" diameter of A1
  measures "d12" diameter of A2
  measures "d13" diameter of A3
  measures "d16" diameter of A4
  measures "d17" distance of L2 L15
  measures "d18" distance of L0 L17
  measures "d26" angle of L5 L6
  measures "d28" distance of P7 P8
  measures "d29" angle of L7 L8
  measures "d31" angle of L9 L10
  measures "d32" distance of P9 P10
  measures "d34" distance of P7 P9
  measures "d43" diameter of A6
  measures "d44" diameter of A7
  measures "d45" diameter of A8
  measures "d46" diameter of A9
  measures "d48" radius of A10
  measures "d49" radius of A11
  measures "d50" radius of A12
  measures "d51" radius of A13
  measures "d65" distance of L19 L20
  measures "d66" distance of L4 L19
  measures "d78" distance of L5 P9
  measures "d79" distance of P7 L36
  measures "d80" distance of P8 L42
  measures "d81" distance of P9 L48
  measures "d82" distance of P10 L54
  measures "d87" distance of P11 L60
  measures "d88" distance of P7 P11
  measures "d91" distance of L67.end L68.end
  measures "d92" distance of L66.end L67.end
  measures "d93" distance of L72.start L72.end
  measures "d94" distance of L72.start L74.end
  measures "d95" distance of L67 L75
  measures "d96" distance of L76.start L76.end
  measures "d97" distance of L3 L80
  measures "d98" distance of L2 L74
  measures "d99" distance of L72 L78
  measures "d100" distance of L76 L78
extrude "Extrude1" add sketch "Sketch1" along normal blind 14 contours A0 | A0 A1 A16 A26 A28 A30 L21 L22 L23 L27 L28 L31 L32 L33 L36 L45 L46 L47 L48 L55 L56 L57 L60 L64 L88 L89 L93 L106 L107 L108 L339 L340 L344 L345 L346 L347 L348 L349 L350 L351 L358 L362 L497 L498 L499 L500 L501 L513 L514 L516 L517 L519 L561 L562 L563 L565 L566 L567 L575 L576 L577 L578 L579 L580 L581 L582 L583 L584 L590 L592 L593 L597 L598 L599 L600 L748 L749 L750 L751 L752 L760 L761 L762 L763 L764 L765 L767 L768 L771 L772 L773 L774 L797 L798 L799 L811 L812 L813 | A0 L15 L27 L501 | A0 L57 L61 L64 | L15 L27 L497 L501 | L57 L60 L61 L64 | L15 L27 L497 L503 L504 L505 L514 | L33 L60 L61 L64 | L15 L27 L514 L516 | L33 L36 L61 L64 | L15 L503 L504 L505 | L15 L27 L516 L738 L739 L740 L748 | L36 L48 L61 L64 | A5 L15 L27 L748 | L45 L48 L61 L64 | A5 L27 | A5 L27 | L15 L738 L739 L740 | A1 L45 L61 L64 | A5 L15 L27 L752 | A1 | L15 A16 L27 L752 L753 L757 L758 L759 | L15 L753 L757 L759 | A16 A17 L27 L758 L761 L767 | A16 L27 L758 | A1 L18 L28 L92 | L15 A16 L758 | A16 A17 L758 L767 | A16 L761 | L18 L28 L90 L92 | L18 L28 L90 L99 L100 L104 L105 | L13 A16 L21 L768 | A16 L21 L767 L768 | L18 L99 L100 L104 | L18 L28 L105 L109 | L13 L21 L768 L771 | L18 L28 L109 L110 L118 L122 L340 L341 | L13 L21 L771 L774 | L18 A14 L28 L340 L341 | L13 L21 L563 L774 | A14 L28 | A14 L28 | L18 L110 L118 L122 | L13 L20 A10 L21 A36 L22 L563 L565 | L18 A14 L28 L343 L344 | L18 A26 L28 L343 L344 L352 L353 L357 L359 | L18 L352 L353 L357 | A26 L28 L350 L359 | A26 A27 L28 L349 L350 | L20 L22 L565 L566 | A26 L349 | A26 L28 L350 L359 | L18 A26 L359 | A26 A27 L28 L350 | L20 L22 L566 L578 | L18 A26 L28 L361 L362 | L20 L22 L578 L797 | L18 A28 L28 L361 L362 L370 L371 | L20 L22 L797 L799 | L18 A28 L370 L371 | A28 L28 L371 L372 L596 L597 | A28 A29 L28 L582 L583 L597 | L20 L22 L799 L813 | L18 A28 L372 | A28 L371 L372 | A28 A29 L582 L583 | A28 L28 L597 | A28 L28 L596 L597 | L12 L20 A13 L22 A37 L23 L811 L813 | L18 A28 L372 L596 | L18 A28 L28 L593 L594 L596 | L18 A30 L28 L593 L594 L603 L604 | A30 A31 L600 L603 | L12 L23 L598 L811 | L18 A30 L603 L604 | A30 A31 L600 | A30 L603 | L12 A30 L23 L598 makes body 1
extrude "Extrude2" add sketch "Sketch1" along normal blind 14 separate body contours L19 A11 L25 L796 L800 | A11 A38 L25 L786 L796 | L19 L25 L800 L801 | L11 A11 L24 A38 L784 L786 | A2 A3 A18 A20 A22 A24 A32 A34 L24 A38 L25 A39 L26 L29 L30 L63 L780 L781 L783 L784 L785 L786 L795 L796 L800 L801 L802 L803 L804 L805 L806 L814 L817 L818 L823 L824 L825 L826 L827 L828 L829 L831 L832 L833 L834 L835 L837 L843 L844 L848 L849 L850 L851 L852 L853 L854 L855 L862 L866 L1001 L1002 L1003 L1004 L1011 L1012 L1013 L1014 L1015 L1016 L1017 L1018 L1021 L1022 L1023 L1030 L1031 L1032 L1033 L1034 L1096 L1097 L1101 L1114 L1115 L1116 L1252 L1253 L1254 L1255 L1262 L1264 L1265 L1266 L1267 L1268 L1269 L1271 L1272 L1273 L1274 L1329 L1330 L1340 L1341 L1505 L1506 L1507 L1508 L1509 L1521 L1522 L1525 L1526 L1527 L1535 L1540 L1541 | L19 L25 L801 L805 | L19 L25 L805 L806 | L11 L24 L783 L784 | L19 A12 L25 A39 L806 L817 | L11 A18 L24 L783 | A18 A19 L779 L780 | L14 A12 A39 L817 L826 | A18 A19 L779 L780 L990 L991 L1004 L1005 | A18 L990 L991 | L14 A39 L26 L825 L826 | L16 A18 L991 | A18 L30 L1004 L1005 | L14 L26 L824 L825 | L16 A18 L991 L1005 | L14 L26 L823 L824 | L16 A18 L30 L1001 L1005 | A18 L30 L1005 | L14 L26 L823 L837 | L26 L823 L824 | L16 A20 L30 L1001 L1007 L1008 | L14 A32 L26 L836 L837 | L16 A20 L1007 L1008 | A20 A21 L30 L1011 | A20 L30 L1008 | L14 A32 L612 L836 | L16 A20 L1008 L1009 | A20 L1008 | A20 A21 L1011 | L16 A20 L30 L1008 L1009 L1018 | L14 A32 L612 | A32 A33 L612 L613 L614 L622 L835 L836 | A32 L26 L836 | A32 A33 L26 L835 L836 | L16 A22 L30 L1018 L1020 | A32 L612 L613 | A22 L30 L1020 L1021 | A22 L30 L1020 | L16 A22 L1020 L1244 | A22 L30 L1020 L1243 L1244 | A22 A23 L30 L1020 L1021 L1022 L1030 | A32 L614 L622 | L17 A32 L29 L622 L626 L844 L845 | L16 A22 L1244 | A22 L1243 L1244 | A22 A23 L1022 L1030 | L16 A22 L30 L1242 L1243 L1252 | L17 A32 L622 L626 | L17 A34 L29 L844 L845 | L16 A22 L1242 L1243 | L16 A24 L30 L1252 | A34 L29 L847 L848 | A34 A35 L29 L848 | A24 A25 L30 L1255 L1256 | A24 L30 L1256 | A34 A35 L29 L848 L849 | L17 A34 L847 | A34 L29 L847 L848 | L16 A24 L1256 | A24 A25 L30 L1255 L1256 L1269 | A24 L30 L1256 | A34 L849 | L17 A34 L29 L847 L854 L856 L857 L861 L863 | L16 A24 L30 L1256 L1257 L1261 L1262 L1263 | A24 L1269 | L17 L856 L857 L861 | L17 L29 L854 L863 L865 L866 | L16 L1257 L1261 L1263 | L16 L30 L1262 L1274 | L17 L29 L865 L866 L874 L875 L876 L1100 L1101 | L16 L30 L1274 L1493 L1494 L1495 L1509 | L17 L29 L1097 L1098 L1100 L1101 | L16 L30 L1505 L1509 | L17 L29 L1097 L1098 L1107 L1108 L1112 L1113 L1114 | L16 L30 L1505 L1511 L1512 L1513 L1522 | L16 L1493 L1494 L1495 | L17 L874 L875 L876 | A3 L17 L29 L1113 L1114 L1117 | A2 L16 L30 L1522 L1524 | A3 L29 L1116 L1117 | A3 L29 L1116 | A2 L30 L1524 L1525 | A2 L30 L1524 | L16 L1511 L1512 L1513 | A3 A8 L1116 L1117 L1118 L1126 L1130 L1338 L1339 L1340 | A3 L17 L1117 | L17 L1107 L1108 L1112 | A2 L16 L1524 | A2 A9 L1524 L1525 L1526 L1534 L1538 | A3 A8 L62 L1339 L1340 | A2 A9 L62 L1526 L1534 | A3 L62 L63 L1336 L1341 | A3 L1118 L1126 L1130 | A2 L62 L63 L1535 L1536 | A3 A8 L62 L1338 L1339 | L62 L63 L1329 L1335 L1336 L1341 | A2 A9 L62 L1534 L1538 | L62 L63 L1535 L1536 L1539 L1540 | L62 L63 L1329 L1330 L1331 L1335 | L62 L63 L1539 L1540 L1541 L1542 | L62 L63 L1330 L1331 L1541 L1542 makes body 2
equation "d18 = d17"
equation "d26 = ( ( 360 / 6 ) / 2 ) * 1 deg"
equation "d28 = ( 12 * 2 ) * 1 mm + 3 mm"
equation "d29 = 180 deg - d26"
equation "d31 = d26"
equation "d32 = d28"
equation "d66 = d65 / 2"
equation "d85 = ( 12 * 4 ) * 1 mm + ( 3 * 2 ) * 1 mm"
equation "d86 = ( 23.38 * 2 ) * 1 mm"
equation "d88 = d34"
equation "d96 = d93 * 6"
equation "d97 = d1 / 2"
